clutch v1 (Autodesk Fusion 360 design; units mm, degrees)
Autodesk Fusion 360 part; units mm, degrees
note: some values were not read from the file. Chosen so that the rebuilt part matches the saved one: which bodies a step acts on.
sketch "Sketch1" plane through (0, 0, 0) normal (0, 1, 0) x (1, 0, 0)
  circle A0 centre (0, 0) radius 12.5
  circle A1 centre (0, 0) radius 25
  constraint coincident A0.centre A1.centre
extrude "Extrude1" add sketch "Sketch1" along normal blind 16 makes body 1
sketch "Sketch2" plane through (0, 0, 0) normal (0, 0, 1) x (1, 0, 0)
  line L0 (0, 0) -> (0, 16)
  line L1 (0, 16) -> (25, 16)
  line L2 (25, 16) -> (25, 8)
  circle A0 centre (18.75, 8) radius 4
  line L3 (-25, 16) -> (-25, 8)
  line L4 (-12.5, 8) -> (-18.75, 8)
  circle A1 centre (-18.75, 8) radius 4
  dimension "d7" = 8
  dimension "d8" = 12.5
  constraint coincident L0.start origin
  constraint vertical L0
  constraint perpendicular L0 L1
  constraint perpendicular L1 L2
  constraint vertical L3
  constraint coincident L4.end A1.centre
  measures "d7" distance of L3.start L3.end
  measures "d8" distance of L3.end L4.start
extrude "Extrude2" add sketch "Sketch2" along normal blind 55 separate body makes body 2 at (-14.7699, 7.6017, 18.3333) makes body 3 at (22.7301, 7.6017, 18.3333)
extrude "Extrude3" add 2 faces at (-17.5044, 7.2272, 0) (19.9513, 7.4215, 0) along direction (0, 0, -1) blind 55 on bodies 2 3 bodies 2 3
combine "Combine1" operation cut target body 1 tool bodies 2 3
sketch "Sketch3" plane through (0, 0, 0) normal (0, 0, 1) x (1, 0, 0)
  line L0 (50, 50) -> (-60, 50)
  line L1 (-60, 50) -> (-60, -55)
  line L2 (-60, -55) -> (50, -55)
  line L3 (50, -55) -> (50, 50)
  constraint horizontal L0
  constraint vertical L1
  constraint horizontal L2
  constraint vertical L3
extrude "Extrude4" cut sketch "Sketch3" along normal blind 0.5 bodies 1 makes body 4 at (-10.2822, 10.6667, -22.7876)
extrude "Extrude5" cut sketch "Sketch3" against normal blind 0.5 bodies 4
sketch "Sketch4" plane through (0, 0, 0) normal (0, -1, 0) x (1, 0, 0)
  line L0 (-12.49, -0.5) -> (-24.995, -0.5)
  arc A0 (-24.995, -0.5) -> (24.995, -0.5) centre (0, 0) ccw
  line L1 (24.995, -0.5) -> (12.49, -0.5)
  arc A1 (-12.49, -0.5) -> (12.49, -0.5) centre (0, 0) ccw
  line L2 (0, 0) -> (-24.995, -0.5)
  line L3 (-24.995, -0.5) -> (-18.7425, -0.5)
  constraint coincident A0.centre A1.centre
  constraint coincident L0.end A0.start
  constraint midpoint L0 L3.end
